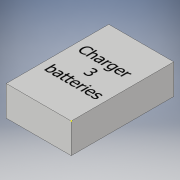
# Autodesk Inventor part: battery charger 2019
Saved by Autodesk Inventor 2019 (Build 230136000, 136)
## iProperties
Created: 2018-12-09
Part Number: battery charger 2019
Material: Generic
Document SubType Name: Modeling
Designer: Tiberus
Density: 1 g/cm^3
Appearance: Default
Author: Tiberus
Autodesk Inventor part; units mm, degrees
ref_plane "YZ Plane" through (0, 0, 0) normal (1, 0, 0) x (0, 1, 0)
ref_plane "XZ Plane" through (0, 0, 0) normal (0, 1, 0) x (-1, 0, 0)
ref_plane "XY Plane" through (0, 0, 0) normal (0, 0, 1) x (1, 0, 0)
sketch "Sketch1" plane through (0, 0, 0) normal (0, 1, 0) x (-1, 0, 0)
  line L0 (0, 0) -> (165.1, 0)
  line L1 (165.1, 0) -> (165.1, -260.35)
  line L2 (165.1, -260.35) -> (0, -260.35)
  line L3 (0, -260.35) -> (0, 0)
  dimension "d0" = 165.1
  dimension "d1" = 260.35
  constraints: 8 end point, 2 parallel, 1 horizontal, 1 perpendicular
  measures "d0" distance of L1.end L2.end
  measures "d1" distance of L0.end L1.end
extrude "Extrusion1" add sketch "Sketch1" along normal blind 76.2
sketch "Sketch2" plane through (0, 76.2, 0) normal (0, 1, 0) x (1, 0, 0)
  line L0 (-163.5139, 239.47) -> (-0.9669, 239.47) construction
  line L1 (-0.9669, 239.47) -> (-0.9669, 25.7814) construction
  line L2 (-0.9669, 25.7814) -> (-163.5139, 25.7814) construction
  line L3 (-163.5139, 25.7814) -> (-163.5139, 239.47) construction
  point P0 (0, 0)
  constraints: 2 other
body "Solid1"
